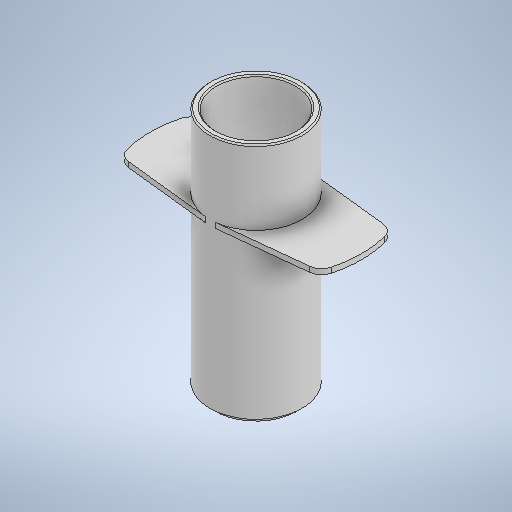
# Autodesk Inventor part: Cylinder
Saved by Autodesk Inventor 2025.2 (Build 292293000, 293)
## iProperties
Created: 2025-06-23
Part Number: Cylinder
Material: Generic
Document SubType Name: Modeling
Designer: Simon
Density: 1 g/cm^3
Appearance: Default
Author: Simon
Autodesk Inventor part; units mm, degrees
ref_plane "YZ Plane" through (0, 0, 0) normal (1, 0, 0) x (0, 1, 0)
ref_plane "XZ Plane" through (0, 0, 0) normal (0, 1, 0) x (-1, 0, 0)
ref_plane "XY Plane" through (0, 0, 0) normal (0, 0, 1) x (1, 0, 0)
sketch "Sketch1" plane through (0, 0, 0) normal (0, 1, 0) x (-1, 0, 0)
  circle A0 centre (0, 0) radius 3
  circle A1 centre (0, 0) radius 1
  dimension "d0" = 6
  dimension "d1" = 2
  constraints: 2 centre point, 2 coincident
  measures "d0" diameter of A0
  measures "d1" diameter of A1
extrude "Extrusion1" add sketch "Sketch1" along normal blind 5.5
sketch "Sketch2" plane through (0, 5.5, 0) normal (0, 1, 0) x (1, 0, 0)
  circle A0 centre (0, 0) radius 1 projected
  circle A1 centre (0, 0) radius 17.5
  dimension "d5" = 35
  constraints: 1 centre point
  measures "d5" diameter of A1
extrude "Extrusion2" add sketch "Sketch2" along normal blind 2
sketch "Sketch3" plane through (0, 7.5, 0) normal (0, 1, 0) x (1, 0, 0)
  circle A0 centre (0, 0) radius 17.5
  circle A1 centre (0, 0) radius 1 projected
  circle A2 centre (0, 0) radius 15
  dimension "d8" = 30
  constraints: 2 centre point, 2 coincident
  measures "d8" diameter of A2
extrude "Extrusion3" add sketch "Sketch3" along normal blind 60 contours A0
thread "Thread1" size "M6x1" class "6g" standard "ISO Metric profile" full length
chamfer "Chamfer1" distance 0.5 angle 45 1 edges at (3, 0, 0)
chamfer "Chamfer2" distance 2 angle 45 1 edges at (-17.5, 5.5, 0)
sketch "Sketch4" plane through (0, 67.5, 0) normal (0, 1, 0) x (1, 0, 0)
  circle A0 centre (0, 0) radius 1 projected
  circle A1 centre (0, 0) radius 15
  circle A2 centre (0, 0) radius 40
  dimension "d19" = 80
  dimension "d25" = 30
  constraints: 2 centre point, 2 coincident
  measures "d19" diameter of A2
  measures "d25" diameter of A1
extrude "Extrusion4" add sketch "Sketch4" along normal blind 2 contours A2
sketch "Sketch5" plane through (0, 69.5, 0) normal (0, 1, 0) x (1, 0, 0)
  circle A0 centre (0, 0) radius 1 projected
  circle A1 centre (0, 0) radius 15
  circle A2 centre (0, 0) radius 17.5
  dimension "d22" = 35
  constraints: 2 centre point, 2 coincident
  measures "d22" diameter of A2
extrude "Extrusion5" add sketch "Sketch5" along normal blind 28 contours A2
sketch "Sketch6" plane through (0, 69.5, 0) normal (0, 1, 0) x (1, 0, 0)
  circle A0 centre (0, 0) radius 1 projected
  circle A1 centre (0, 0) radius 17.5
  circle A2 centre (0, 0) radius 3 projected
  circle A3 centre (0, 0) radius 50
  circle A4 centre (-50, 0) radius 12.5
  line L0 (-48.4375, -12.402) -> (-1.8675, -17.4001)
  line L1 (-48.4375, 12.402) -> (-1.8675, 17.4001)
  circle A5 centre (0, 0) radius 17.5 projected
  line L2 (50, 0) -> (-50, 0)
  circle A6 centre (50, 0) radius 12.5
  line L3 (48.4375, -12.402) -> (1.8675, -17.4001)
  line L4 (48.4375, 12.402) -> (1.8675, 17.4001)
  point P0 (1.8675, 17.4001)
  point P1 (1.8675, -17.4001)
  dimension "d26" = 35
  dimension "d27" = 100
  dimension "d29" = 25
  dimension "d30" = 25
  constraints: 13 point on circle, 10 end point, 4 centre point, 4 tangent, 3 coincident, 1 horizontal, 1 midpoint
  measures "d26" diameter of A1
  measures "d27" diameter of A3
  measures "d29" diameter of A4
  measures "d30" diameter of A6
extrude "Extrusion6" cut sketch "Sketch6" against normal through all contours A1 L1 A3 L4 | L3 A3 L0 A1
fillet "Fillet1" radius 5 4 edges at (-37.6308, 68.5, 13.5618) (37.6308, 68.5, 13.5618) (37.6308, 68.5, -13.5618) (-37.6308, 68.5, -13.5618)
chamfer "Chamfer3" distance 0.5 angle 45 1 edges at (-17.5, 97.5, 0)
chamfer "Chamfer4" distance 0.5 angle 45 1 edges at (-15, 97.5, 0)
body "Solid1"
